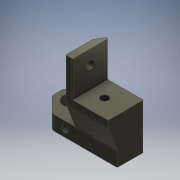
# Autodesk Inventor part: Z Axis Linear Rail Bracket - Double Z - Left 1.0
Saved by Autodesk Inventor 2016 (Build 200138000, 138)
## iProperties
Created: 2017-02-13
Part Number: Z Axis Linear Rail Bracket - Double Z - Left 1.0
Material: PC/ABS Plastic
Document SubType Name: Modeling
Designer: Scott
Density: 0.357273 g/cm^3
Appearance: Gunmetal
Author: Scott
Autodesk Inventor part; units mm, degrees
sketch "Sketch1" plane through (0, 0, 0) normal (0, 0, 1) x (1, 0, 0)
  circle A0 centre (0, 0) radius 6
  line L0 (0, 0) -> (83.2978, 0) construction
  circle A1 centre (37, 0) radius 2.6
  line L1 (-10, 10) -> (47, 10)
  line L2 (47, 10) -> (47, -15)
  line L3 (47, -15) -> (-10, -15)
  line L4 (-10, -15) -> (-10, 10)
  line L5 (22, 29.5766) -> (22, -18.8569) construction
  dimension "d0" = 12
  dimension "d1" = 5.2
  dimension "d2" = 37
  dimension "d3" = 10
  dimension "d4" = 15
  dimension "d5" = 10
  dimension "d6" = 22
  dimension "d7" = 25
  constraints: 12 end point, 3 perpendicular, 2 centre point, 2 horizontal, 1 coincident, 1 point on line, 1 vertical
  measures "d0" diameter of A0
  measures "d1" diameter of A1
  measures "d2" distance of A1.centre L0.start
  measures "d3" distance between parallel lines of L0 L1
  measures "d4" distance between parallel lines of L0 L3
  measures "d5" distance from line of L4 L0.start
  measures "d6" distance from line of L0.start L5
  measures "d7" distance between parallel lines of L2 L5
extrude "Extrusion1" add sketch "Sketch1" along normal blind 5 contours A1 | L1 L2 L3 L4
sketch "Sketch2" plane through (0, 0, 5) normal (0, 0, 1) x (1, 0, 0)
  circle A0 centre (0, 0) radius 6 projected
  line L0 (47, 10) -> (-10, 10) projected
  line L1 (-10, 10) -> (-10, -15) projected
  line L2 (-10, -15) -> (47, -15) projected
  line L3 (47, -15) -> (47, 10) projected
  line L4 (22, 10) -> (22, -15)
  dimension "d10" = 22
  constraints: 2 end point, 2 point on line, 1 perpendicular
  measures "d10" distance from line of L4 A0.centre
extrude "Extrusion2" add sketch "Sketch2" along normal blind 5 contours L4 L2 L1 L0
sketch "Sketch4" plane through (0, 0, 5) normal (0, 0, 1) x (1, 0, 0)
  circle A0 centre (0, 0) radius 6 projected
  line L0 (-10, 10) -> (-10, -15) projected
  line L1 (-10, -15) -> (22, -15) projected
  line L2 (22, -15) -> (22, 10) projected
  line L3 (22, 10) -> (-10, 10) projected
  line L4 (22, 10) -> (17, 10)
  line L5 (17, 10) -> (17, -15)
  line L6 (17, -15) -> (22, -15)
  line L7 (22, -15) -> (22, 10)
  dimension "d13" = 5
  constraints: 8 end point, 2 parallel, 1 horizontal, 1 perpendicular, 1 point on line
  measures "d13" distance between parallel lines of L5 L2
extrude "Extrusion3" add sketch "Sketch4" along normal blind 25 contours L3 L2 L1 L5
chamfer "Chamfer1" distance 6 angle 45 1 edges at (-10, 10, 5)
chamfer "Chamfer2" distance 2 angle 45 1 edges at (17, -2.5, 10)
chamfer "Chamfer3" distance 11 angle 45 1 edges at (-10, -15, 5)
sketch "Sketch7" plane through (0, 0, 10) normal (0, 0, 1) x (1, 0, 0)
  line L0 (15, 10) -> (15, -15) projected
  line L1 (15, 10) -> (-4, 10) projected
  line L2 (-10, 4) -> (-4, 10) projected
  line L3 (-10, 4) -> (-10, -4) projected
  line L4 (1, -15) -> (15, -15) projected
  circle A0 centre (0, 0) radius 6 projected
  line L5 (14.25, 10) -> (14.25, 4.25)
  line L6 (14.25, 4.25) -> (4.2353, 4.25)
  line L7 (4.8734, 3.5) -> (15, 3.5)
  line L8 (1, -15) -> (-10, -4) projected
  dimension "d33" = 0.75
  dimension "d34" = 0.75
  dimension "d35" = 3.5
  constraints: 6 end point, 2 point on circle, 2 point on line, 1 horizontal, 1 perpendicular, 1 vertical
  measures "d33" distance between parallel lines of L0 L5
  measures "d34" distance between parallel lines of L6 L7
  measures "d35" distance from line of point (0, 0) L7
extrude "Extrusion5" cut sketch "Sketch7" against normal through all contours L0 L7 A0 L6 L5 L1
fillet "Fillet1" radius 0.5 1 edges at (4.8734, 3.5, 5)
fillet "Fillet2" radius 0.5 1 edges at (4.2353, 4.25, 5)
sketch "Sketch8" plane through (-4, 10, 10) normal (0, 1, 0) x (1, 0, 0)
  line L0 (18.25, 0) -> (18.25, 10) projected
  line L1 (0, 10) -> (18.25, 10) projected
  line L2 (0, 0) -> (0, 10) projected
  line L3 (18.25, 0) -> (0, 0) projected
  point P0 (4, 10)
  point P1 (14, 5)
  dimension "d40" = 10
  dimension "d41" = 5
  measures "d40" horizontal distance of point (4, 10) point (14, 5)
  measures "d41" distance from line of L1 point (14, 5)
hole "Hole2" at (10, 10, 5) direction (0, -1, 0) diameter 3.5 end through all
sketch "Sketch9" plane through (47, -15, 0) normal (0, -1, 0) x (1, 0, 0)
  circle A0 centre (-37, 5) radius 1.75 projected
  circle A1 centre (-37, 5) radius 1.75 projected
  point P0 (-47, 0)
  constraints: 1 coincident
hole "Hole3" at (10, -15, 5) direction (0, 1, 0) diameter 4.7 depth 5 counterbore diameter 5 counterbore depth 0.5
fillet "Fillet5" radius 4 4 edges at (-4, 10, 5) (-10, 4, 5) (-10, -4, 5) (1, -15, 5)
sketch "Sketch10" plane through (0, 0, 10) normal (0, 0, 1) x (1, 0, 0)
  line L0 (-10, 10) -> (47, 10)
  line L1 (47, 10) -> (47, -15)
  line L2 (47, -15) -> (-10, -15)
  line L3 (-10, -15) -> (-10, 10)
  line L4 (14.25, 10) -> (-2.3431, 10) projected
  line L5 (-10, 2.3431) -> (-10, -2.3431) projected
  line L6 (2.6569, -15) -> (15, -15) projected
  line L7 (47, -15) -> (47, 10) projected
  point P0 (0, 0)
  constraints: 8 end point, 4 collinear, 2 parallel, 1 horizontal, 1 perpendicular
extrude "Extrusion6" cut sketch "Sketch10" along normal through all
sketch "Sketch11" plane through (0, 0, 10) normal (0, 0, 1) x (1, 0, 0)
  line L0 (14.25, 4.25) -> (14.25, 10) projected
  line L1 (15, 3.5) -> (5.7663, 3.5) projected
  line L2 (14.25, 10) -> (47, 10)
  line L3 (47, 10) -> (47, 3.5)
  line L4 (47, 3.5) -> (14.25, 3.5)
  line L5 (14.25, 3.5) -> (14.25, 10)
  line L6 (15, 10) -> (22, 10) projected
  line L7 (47, -15) -> (47, 10) projected
  point P0 (0, 0)
  constraints: 8 end point, 4 collinear, 2 parallel, 1 horizontal, 1 perpendicular
extrude "Extrusion7" cut sketch "Sketch11" against normal through all
sketch "Sketch12" plane through (0, 0, 5) normal (0, 0, 1) x (1, 0, 0)
  line L0 (47, 3.5) -> (22, 3.5) projected
  line L1 (22, 3.5) -> (22, -15) projected
  line L2 (22, -15) -> (47, -15) projected
  line L3 (47, -15) -> (47, 3.5) projected
  point P0 (0, 0)
extrude "Extrusion8" add sketch "Sketch12" along normal up to surface (5 mm away)
ref_plane "Work Plane1" through (0, 0, 0) normal (-1, 0, 0) x (0, 0, 1)
ref_plane "Work Plane2" through (17, 0, 0) normal (-1, 0, 0) x (0, 0, 1)
sketch "Sketch13" plane through (17, 0, 0) normal (-1, 0, 0) x (0, 0, 1)
  line L0 (57, 3.5) -> (57, -21.5)
  line L1 (57, -21.5) -> (27, -21.5)
  line L2 (0, 3.5) -> (0, -15) projected
  line L3 (57, 3.5) -> (0, 3.5)
  line L4 (27, -21.5) -> (10, -15)
  line L5 (0, -15) -> (10, -15) projected
  line L6 (10, -15) -> (0, -15)
  line L7 (0, -15) -> (0, 3.5)
  point P0 (0, 0)
  point P1 (10, 3.5)
  dimension "d72" = 30
  dimension "d73" = 25
  dimension "d83" = 27
  constraints: 12 end point, 2 perpendicular, 1 collinear, 1 horizontal, 1 parallel
  measures "d72" distance of L0.end L1.end
  measures "d73" distance of L0.start L0.end
  measures "d83" distance from line of L1.end L2
extrude "Extrusion9" add sketch "Sketch13" against normal up to surface (30 mm away)
ref_plane "Work Plane3" through (22, 0, 0) normal (-1, 0, 0) x (0, 0, 1)
sketch "Sketch14" plane through (22, 0, 0) normal (-1, 0, 0) x (0, 0, 1)
  line L0 (10, -15) -> (10, 3.5) projected
  line L1 (27, -21.5) -> (57, -21.5) projected
  line L2 (57, -21.5) -> (57, 3.5) projected
  line L3 (57, 3.5) -> (32, 3.5)
  line L4 (32, 3.5) -> (32, -21.5)
  line L5 (32, -21.5) -> (57, -21.5)
  line L6 (57, -21.5) -> (57, 3.5)
  line L7 (57, 3.5) -> (10, 3.5) projected
  line L8 (10, -15) -> (27, -21.5) projected
  point P0 (0, 0)
  dimension "d77" = 25
  constraints: 8 end point, 2 parallel, 1 horizontal, 1 perpendicular, 1 point on line
  measures "d77" distance between parallel lines of L4 L2
extrude "Extrusion10" cut sketch "Sketch14" against normal through all contours L3 L2 L1 L4
chamfer "Chamfer5" distance 6 angle 30 1 edges at (17, 3.5, 33.5) measured on face at (17, 3, 33.5)
chamfer "Chamfer6" distance 1.5 angle 45 1 edges at (14.25, 10, 5)
sketch "Sketch15" plane through (0, 0, 0) normal (0, 0, -1) x (-1, 0, 0)
  line L0 (-14.25, 8.5) -> (-12.75, 10) projected
  line L1 (-14.25, 8.5) -> (-14.25, 4.25) projected
  line L2 (-14.25, 4.25) -> (-4.4371, 4.25) projected
  arc A0 (-4.4371, 4.25) -> (-4.0957, 4.3846) centre (-4.4371, 4.75) ccw projected
  arc A1 (-5.3227, 2.7692) -> (-4.0957, 4.3846) centre (0, 0) ccw projected
  arc A2 (-5.3227, 2.7692) -> (-5.7663, 3.5) centre (-5.7663, 3) ccw projected
  line L3 (-5.7663, 3.5) -> (-47, 3.5) projected
  line L4 (-47, 3.5) -> (-47, -15) projected
  line L5 (-47, -15) -> (-2.6569, -15) projected
  arc A3 (-2.6569, -15) -> (0.1716, -13.8284) centre (-2.6569, -11) ccw projected
  line L6 (8.8284, -5.1716) -> (0.1716, -13.8284) projected
  arc A4 (8.8284, -5.1716) -> (10, -2.3431) centre (6, -2.3431) ccw projected
  line L7 (10, -2.3431) -> (10, 2.3431) projected
  arc A5 (10, 2.3431) -> (8.8284, 5.1716) centre (6, 2.3431) ccw projected
  line L8 (5.1716, 8.8284) -> (8.8284, 5.1716) projected
  arc A6 (5.1716, 8.8284) -> (2.3431, 10) centre (2.3431, 6) ccw projected
  line L9 (2.3431, 10) -> (-12.75, 10) projected
  line L10 (-20.4641, 3.5) -> (-5.7663, 3.5) projected
  line L11 (-15, 3.5) -> (-15, 7.75)
  line L12 (-15, 7.75) -> (-19.25, 3.5)
  line L13 (-5.7663, 3.5) -> (-47, 3.5) projected
  line L14 (-19.25, 3.5) -> (-15, 3.5)
  line L15 (-14.25, 8.5) -> (-12.75, 10) projected
  dimension "d90" = 0.75
  constraints: 6 end point, 2 collinear, 2 point on line, 1 perpendicular
  measures "d90" distance between parallel lines of L11 L1
extrude "Extrusion11" add sketch "Sketch15" against normal blind 10 contours L3 L12 L11
fillet "Fillet6" radius 0.5 3 edges at (15, 7.75, 5) (14.25, 8.5, 5) (12.75, 10, 5)
fillet "Fillet7" radius 5 2 edges at (32, -15, 10) (32, -21.5, 27)
fillet "Fillet8" radius 0.5 14 edges at (17, -21.4169, 27.0153) (17, -21.5, 42.4616) (17, -15.0831, 9.9847) (17, -18.25, 18.5) (17, -2.5, 33.5) (47, -21.4169, 27.0153) (47, -21.5, 29.9616) (47, -15.0831, 9.9847) (47, -15, 4.5384) (47, -18.25, 18.5) (47, 3.5, 16) (20.4641, 3.5, 33.5) (22, -21.5, 44.5) (22, 3.5, 44.5)
fillet "Fillet9" radius 3 1 edges at (19.25, 3.5, 5)
sketch "Sketch16" plane through (0, 0, 0) normal (0, 0, -1) x (-1, 0, 0)
  line L0 (-46.5, -21.5) -> (-17.5, -21.5) projected
  line L1 (-47, -14.8627) -> (-47, -20.7032) projected
  point P0 (0, 0)
  point P1 (-32, -9)
  dimension "d97" = 15
  dimension "d98" = 12.5
  measures "d97" distance from line of point (-32, -9) L1
  measures "d98" distance from line of point (-32, -9) L0
hole "Hole4" at (32, -9, 0) direction (0, 0, 1) diameter 5.4 end through all
ref_plane "Work Plane4" through (22, -21, 27) normal (0, 0, 1) x (1, 0, 0)
hole "Hole5" at (32, -9, 0) direction (0, 0, 1) diameter 10.5 depth 27
sketch "Sketch17" plane through (32, -9, 27) normal (0, 0, -1) x (-1, 0, 0)
  circle A0 centre (0, 0) radius 2.7 projected
  point P0 (32, 9)
extrude "Extrusion12" add sketch "Sketch17" against normal blind 0.4
sketch "Sketch18" plane through (17, 0, 0) normal (-1, 0, 0) x (0, 0, 1)
  line L0 (27.9233, -21.5) -> (57, -21.5) projected
  line L1 (57, -21) -> (57, -2.634) projected
  circle A0 centre (47, -9) radius 2.7
  line L2 (32, 3) -> (32, -21) projected
  point P0 (0, 0)
  dimension "d119" = 12.5
  dimension "d120" = 15
  dimension "d121" = 5.4
  constraints: 1 centre point
  measures "d119" distance from line of L0 A0.centre
  measures "d120" distance from line of A0.centre L2
  measures "d121" diameter of A0
extrude "Extrusion13" cut sketch "Sketch18" against normal through all
body "Solid1"
